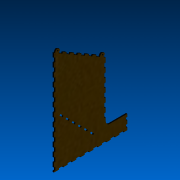
# Autodesk Inventor part: cote
Saved by Autodesk Inventor 2013 SP2 (Build 170200200, 200)
## iProperties
Created: 2015-09-15
Part Number: cote
Material: Generic
Document SubType Name: Modeling
Designer: jeanfrancois
Density: 1 g/cm^3
Author: jeanfrancois
Autodesk Inventor part; units mm, degrees
ref_plane "YZ Plane" through (0, 0, 0) normal (1, 0, 0) x (0, 1, 0)
ref_plane "XZ Plane" through (0, 0, 0) normal (0, 1, 0) x (-1, 0, 0)
ref_plane "XY Plane" through (0, 0, 0) normal (0, 0, 1) x (1, 0, 0)
sketch "Esquisse1" plane through (0, 0, 0) normal (1, 0, 0) x (0, 1, 0)
  line L0 (86.0493, 43.9619) -> (86.0493, 33.9619)
  line L1 (89.0493, 43.9619) -> (86.0493, 43.9619)
  line L2 (89.0493, 53.9619) -> (89.0493, 43.9619)
  line L3 (89.0493, 53.9619) -> (86.0493, 53.9619)
  line L4 (86.0493, 63.9619) -> (86.0493, 53.9619)
  line L5 (89.0493, 63.9619) -> (86.0493, 63.9619)
  line L6 (89.0493, 73.9619) -> (89.0493, 63.9619)
  line L7 (89.0493, 73.9619) -> (86.0493, 73.9619)
  line L8 (86.0493, 83.9619) -> (86.0493, 73.9619)
  line L9 (89.0493, 83.9619) -> (86.0493, 83.9619)
  line L10 (89.0493, 93.9619) -> (89.0493, 83.9619)
  line L11 (89.0493, 93.9619) -> (86.0493, 93.9619)
  line L12 (89.0493, 103.9619) -> (86.0493, 103.9619)
  line L13 (86.0493, 103.9619) -> (86.0493, 93.9619)
  line L14 (89.0493, 113.9619) -> (89.0493, 103.9619)
  line L15 (83.841, 116.969) -> (89.0493, 113.9619)
  line L16 (86.841, 122.1651) -> (83.841, 116.969)
  line L17 (80.9128, 127.8972) -> (86.1089, 124.8972)
  line L18 (78.1807, 127.1651) -> (75.1807, 121.969)
  line L19 (66.5204, 126.969) -> (75.1807, 121.969)
  line L20 (89.0493, 33.9619) -> (86.0493, 33.9619)
  line L21 (40.5363, -53.7785) -> (50.5363, -53.7785)
  line L22 (50.5363, -56.7785) -> (60.5363, -56.7785)
  line L23 (50.5363, -53.7785) -> (50.5363, -56.7785)
  line L24 (60.5363, -53.7785) -> (60.5363, -56.7785)
  line L25 (60.5363, -53.7785) -> (70.5363, -53.7785)
  line L26 (70.5363, -56.7785) -> (80.5363, -56.7785)
  line L27 (70.5363, -53.7785) -> (70.5363, -56.7785)
  line L28 (80.5363, -53.7785) -> (80.5363, -56.7785)
  line L29 (80.5363, -53.7785) -> (90.5363, -53.7785)
  line L30 (90.5363, -53.7785) -> (90.5363, -56.7785)
  line L31 (139.0363, -30.2785) -> (139.0363, -23.7561)
  line L32 (139.0363, -44.2785) -> (139.0363, -36.2785)
  line L33 (139.0363, -56.7785) -> (139.0363, -50.2785)
  line L34 (136.0363, -36.2785) -> (136.0363, -30.2785)
  line L35 (139.0363, -50.2785) -> (136.0363, -50.2785)
  line L36 (139.0363, -30.2785) -> (136.0363, -30.2785)
  line L37 (139.0363, -44.2785) -> (136.0363, -44.2785)
  line L38 (139.0363, -36.2785) -> (136.0363, -36.2785)
  line L39 (136.0363, -50.2785) -> (136.0363, -44.2785)
  line L40 (130.5363, -53.7785) -> (130.5363, -56.7785)
  line L41 (130.5363, -56.7785) -> (139.0363, -56.7785)
  line L42 (120.5363, -53.7785) -> (120.5363, -56.7785)
  line L43 (110.5363, -53.7785) -> (110.5363, -56.7785)
  line L44 (110.5363, -56.7785) -> (120.5363, -56.7785)
  line L45 (99.0493, -23.7561) -> (139.0363, -23.7561)
  line L46 (100.5363, -53.7785) -> (110.5363, -53.7785)
  line L47 (100.5363, -53.7785) -> (100.5363, -56.7785)
  arc A0 (89.0493, -13.7561) -> (99.0493, -23.7561) centre (99.0493, -13.7561) ccw
  line L48 (90.5363, -56.7785) -> (100.5363, -56.7785)
  line L49 (120.5363, -53.7785) -> (130.5363, -53.7785)
  line L50 (10.2252, 22.79) -> (17.2962, 15.719)
  line L51 (12.3465, 24.9113) -> (19.4175, 17.8403)
  line L52 (26.4886, 10.7692) -> (33.5597, 3.6981)
  line L53 (24.3673, 8.6479) -> (31.4384, 1.5768)
  line L54 (38.5094, -5.4942) -> (45.5805, -12.5653)
  line L55 (40.6307, -3.3729) -> (47.7018, -10.444)
  line L56 (54.7729, -17.5151) -> (61.8439, -24.5861)
  line L57 (52.6516, -19.6364) -> (59.7226, -26.7074)
  line L58 (59.7226, -26.7074) -> (61.8439, -24.5861)
  line L59 (52.6516, -19.6364) -> (54.7729, -17.5151)
  line L60 (45.5805, -12.5653) -> (47.7018, -10.444)
  line L61 (38.5094, -5.4942) -> (40.6307, -3.3729)
  line L62 (31.4384, 1.5768) -> (33.5597, 3.6981)
  line L63 (3.1541, 29.8611) -> (5.2754, 31.9824)
  line L64 (10.2252, 22.79) -> (12.3465, 24.9113)
  line L65 (17.2962, 15.719) -> (19.4175, 17.8403)
  line L66 (24.3673, 8.6479) -> (26.4886, 10.7692)
  line L67 (89.0493, -6.0381) -> (89.0493, -13.7561)
  line L68 (89.0493, -6.0381) -> (86.0493, -6.0381)
  line L69 (86.0493, 3.9619) -> (86.0493, -6.0381)
  line L70 (89.0493, 3.9619) -> (86.0493, 3.9619)
  line L71 (89.0493, 13.9619) -> (89.0493, 3.9619)
  line L72 (89.0493, 13.9619) -> (86.0493, 13.9619)
  line L73 (86.0493, 23.9619) -> (86.0493, 13.9619)
  line L74 (89.0493, 33.9619) -> (89.0493, 23.9619)
  line L75 (89.0493, 23.9619) -> (86.0493, 23.9619)
  line L76 (24.7192, 154.567) -> (33.3794, 149.567)
  line L77 (33.3794, 149.567) -> (31.8794, 146.969)
  line L78 (31.8794, 146.969) -> (40.5397, 141.969)
  line L79 (42.0397, 144.567) -> (40.5397, 141.969)
  line L80 (42.0397, 144.567) -> (50.6999, 139.567)
  line L81 (50.6999, 139.567) -> (49.1999, 136.969)
  line L82 (49.1999, 136.969) -> (57.8602, 131.969)
  line L83 (59.3602, 134.567) -> (57.8602, 131.969)
  line L84 (68.0204, 129.567) -> (66.5204, 126.969)
  line L85 (59.3602, 134.567) -> (68.0204, 129.567)
  line L86 (40.5363, -53.7785) -> (40.5363, -56.7785)
  line L87 (30.5363, -56.7785) -> (40.5363, -56.7785)
  line L88 (30.5363, -53.7785) -> (30.5363, -56.7785)
  line L89 (20.5363, -53.7785) -> (30.5363, -53.7785)
  line L90 (20.5363, -53.7785) -> (20.5363, -56.7785)
  line L91 (10.5363, -56.7785) -> (20.5363, -56.7785)
  line L92 (0.5363, -53.7785) -> (10.5363, -53.7785)
  line L93 (0.5363, -53.7785) -> (0.5363, -56.7785)
  line L94 (-9.4637, -56.7785) -> (0.5363, -56.7785)
  line L95 (10.5363, -53.7785) -> (10.5363, -56.7785)
  line L96 (-30.9637, -56.7785) -> (-19.4637, -56.7785)
  line L97 (-19.4637, -53.7785) -> (-19.4637, -56.7785)
  line L98 (-19.4637, -53.7785) -> (-9.4637, -53.7785)
  line L99 (-9.4637, -53.7785) -> (-9.4637, -56.7785)
  line L100 (-1.7957, 39.0535) -> (5.2754, 31.9824)
  line L101 (-3.917, 36.9322) -> (3.1541, 29.8611)
  line L102 (-18.0591, 51.0743) -> (-15.9378, 53.1956)
  line L103 (-10.988, 44.0032) -> (-8.8667, 46.1246)
  line L104 (-3.917, 36.9322) -> (-1.7957, 39.0535)
  line L105 (-18.0591, 51.0743) -> (-10.988, 44.0032)
  line L106 (-15.9378, 53.1956) -> (-8.8667, 46.1246)
  line L107 (-30.9637, 63.2215) -> (-27.9637, 63.2215)
  line L108 (-27.9637, 73.2215) -> (-27.9637, 63.2215)
  line L109 (-30.9637, 73.2215) -> (-27.9637, 73.2215)
  line L110 (-30.9637, 83.2215) -> (-27.9637, 83.2215)
  line L111 (-27.9637, 93.2215) -> (-27.9637, 83.2215)
  line L112 (-30.9637, 93.2215) -> (-27.9637, 93.2215)
  line L113 (-30.9637, 103.2215) -> (-30.9637, 93.2215)
  line L114 (-30.9637, 103.2215) -> (-27.9637, 103.2215)
  line L115 (-27.9637, 113.2215) -> (-27.9637, 103.2215)
  line L116 (-30.9637, 113.2215) -> (-27.9637, 113.2215)
  line L117 (-30.9637, 83.2215) -> (-30.9637, 73.2215)
  line L118 (-30.9637, 163.2215) -> (-30.9637, 153.2215)
  line L119 (-30.9637, 183.2215) -> (-30.9637, 173.2215)
  line L120 (-30.9637, 183.2215) -> (-28.7553, 181.9465)
  line L121 (-30.9637, 153.2215) -> (-27.9637, 153.2215)
  line L122 (-30.9637, 163.2215) -> (-27.9637, 163.2215)
  line L123 (-27.9637, 173.2215) -> (-27.9637, 163.2215)
  line L124 (-30.9637, 173.2215) -> (-27.9637, 173.2215)
  line L125 (-30.9637, 143.2215) -> (-30.9637, 133.2215)
  line L126 (-30.9637, 143.2215) -> (-27.9637, 143.2215)
  line L127 (-30.9637, 123.2215) -> (-30.9637, 113.2215)
  line L128 (-30.9637, 133.2215) -> (-27.9637, 133.2215)
  line L129 (-30.9637, 123.2215) -> (-27.9637, 123.2215)
  line L130 (-27.9637, 133.2215) -> (-27.9637, 123.2215)
  line L131 (-27.9637, 153.2215) -> (-27.9637, 143.2215)
  line L132 (-25.7423, 187.1651) -> (-28.7553, 181.9465)
  line L133 (-23.0103, 187.8972) -> (-17.8141, 184.8972)
  line L134 (-17.0821, 182.1651) -> (-20.0821, 176.969)
  line L135 (-20.0821, 176.969) -> (-11.4218, 171.969)
  line L136 (-9.9218, 174.567) -> (-11.4218, 171.969)
  line L137 (-9.9218, 174.567) -> (-1.2616, 169.567)
  line L138 (-1.2616, 169.567) -> (-2.7616, 166.969)
  line L139 (-2.7616, 166.969) -> (5.8987, 161.969)
  line L140 (7.3987, 164.567) -> (5.8987, 161.969)
  line L141 (7.3987, 164.567) -> (16.0589, 159.567)
  line L142 (16.0589, 159.567) -> (14.5589, 156.969)
  line L143 (14.5589, 156.969) -> (23.2192, 151.969)
  line L144 (24.7192, 154.567) -> (23.2192, 151.969)
  line L145 (-27.9637, -46.7785) -> (-27.9637, -53.7785)
  line L146 (-30.9637, -36.7785) -> (-30.9637, -46.7785)
  line L147 (-30.9637, -46.7785) -> (-27.9637, -46.7785)
  line L148 (-30.9637, -36.7785) -> (-27.9637, -36.7785)
  line L149 (-30.9637, -16.7785) -> (-30.9637, -26.7785)
  line L150 (-30.9637, -26.7785) -> (-27.9637, -26.7785)
  line L151 (-30.9637, -16.7785) -> (-27.9637, -16.7785)
  line L152 (-30.9637, 3.2215) -> (-30.9637, -6.7785)
  line L153 (-30.9637, -6.7785) -> (-27.9637, -6.7785)
  line L154 (-27.9637, -6.7785) -> (-27.9637, -16.7785)
  line L155 (-27.9637, -26.7785) -> (-27.9637, -36.7785)
  line L156 (-30.9637, 63.2215) -> (-30.9637, 53.2215)
  line L157 (-30.9637, 53.2215) -> (-27.9637, 53.2215)
  line L158 (-27.9637, 53.2215) -> (-27.9637, 43.2215)
  line L159 (-30.9637, 43.2215) -> (-27.9637, 43.2215)
  line L160 (-30.9637, 43.2215) -> (-30.9637, 33.2215)
  line L161 (-30.9637, 33.2215) -> (-27.9637, 33.2215)
  line L162 (-27.9637, 33.2215) -> (-27.9637, 23.2215)
  line L163 (-30.9637, 23.2215) -> (-27.9637, 23.2215)
  line L164 (-30.9637, 23.2215) -> (-30.9637, 13.2215)
  line L165 (-30.9637, 13.2215) -> (-27.9637, 13.2215)
  line L166 (-27.9637, 13.2215) -> (-27.9637, 3.2215)
  line L167 (-30.9637, 3.2215) -> (-27.9637, 3.2215)
  line L168 (-27.9637, -53.7785) -> (-30.9637, -53.7785)
  line L169 (-30.9637, -53.7785) -> (-30.9637, -56.7785)
  line L170 (-25.7423, 187.1651) -> (-23.0103, 187.8972)
  line L171 (-17.8141, 184.8972) -> (-17.0821, 182.1651)
  line L172 (78.1807, 127.1651) -> (80.9128, 127.8972)
  line L173 (86.1089, 124.8972) -> (86.841, 122.1651)
  circle A1 centre (-22.1622, 183.3661) radius 1.5
  circle A2 centre (81.7608, 123.3661) radius 1.5
  point P0 (0, 0)
  point P1 (87.841, 123.8972)
  point P2 (79.1807, 128.8972)
  point P3 (-27.9637, -56.7785)
  point P4 (-24.7423, 188.8972)
  point P5 (-16.0821, 183.8972)
  dimension "d2" = 10
  dimension "d4" = 20
  dimension "d5" = 3
  dimension "d6" = 7
  dimension "d7" = 8
  dimension "d8" = 8
  dimension "d9" = 2
  dimension "d10" = 2
  dimension "d11" = 2
  dimension "d12" = 2
  dimension "d13" = 2
  dimension "d14" = 2
  dimension "d15" = 2
  dimension "d16" = 2
  dimension "d17" = 3
  dimension "d18" = 4.5
  dimension "d19" = 3
  dimension "d20" = 4.5
  constraints: 348 end point, 9 point on line, 3 centre point, 2 point on circle, 1 parallel, 1 perpendicular
  measures "d2" distance of L146.start L146.end
  measures "d4" distance between parallel lines of L96 L148
  measures "d5" distance of L145.end L168.end
  measures "d6" distance between parallel lines of L168 L147
  measures "d7" distance between parallel lines of L17 L15
  measures "d8" distance between parallel lines of L133 L135
  measures "d9" distance of L132.start point (-24.742, 188.897)
  measures "d10" distance of L133.start point (-24.742, 188.897)
  measures "d11" distance of L133.end point (-16.082, 183.897)
  measures "d12" distance of L134.start point (-16.082, 183.897)
  measures "d13" distance of L18.start point (79.181, 128.897)
  measures "d14" distance of L17.start point (79.181, 128.897)
  measures "d15" distance of L17.end point (87.841, 123.897)
  measures "d16" distance of L16.start point (87.841, 123.897)
  measures "d17" diameter of A1
  measures "d18" distance from line of L135 A1.centre
  measures "d19" diameter of A2
  measures "d20" distance from line of A2.centre L19
extrude "Extrusion1" add sketch "Esquisse1" along normal blind 3 contours L0 L20 L74 L75 L73 L72 L71 L70 L69 L68 L67 A0 L45 L31 L36 L34 L38 L32 L37 L39 L35 L33 L41 L40 L49 L42 L44 L43 L46 L47 L48 L30 L29 L28 L26 L27 L25 L24 L22 L23 L21 L86 L87 L88 L89 L90 L91 L95 L92 L93 L94 L99 L98 L97 L96 L169 L168 L145 L147 L146 L148 L155 L150 L149 L151 L154 L153 L152 L167 L166 L165 L164 L163 L162 L161 L160 L159 L158 L157 L156 L107 L108 L109 L117 L110 L111 L112 L113 L114 L115 L116 L127 L129 L130 L128 L125 L126 L131 L121 L118 L122 L123 L124 L119 L120 L132 L170 L133 L171 L134 L135 L136 L137 L138 L139 L140 L141 L142 L143 L144 L76 L77 L78 L79 L80 L81 L82 L83 L85 L84 L19 L18 L172 L17 L173 L16 L15 L14 L12 L13 L11 L10 L9 L8 L7 L6 L5 L4 L3 L2 L1 | A1 | A2
hole "Perçage1" at (3, 81.7608, 123.3661) direction (-1, 0, 0) diameter 3 end through all
hole "Perçage2" at (3, -22.1622, 183.3661) direction (-1, 0, 0) diameter 3 end through all
equation "\"d8\" = d7"
equation "\"d10\" = d9"
equation "\"d11\" = d9"
equation "\"d12\" = d11"
equation "\"d13\" = d9"
equation "\"d14\" = d13"
equation "\"d15\" = d9"
equation "\"d16\" = d15"
